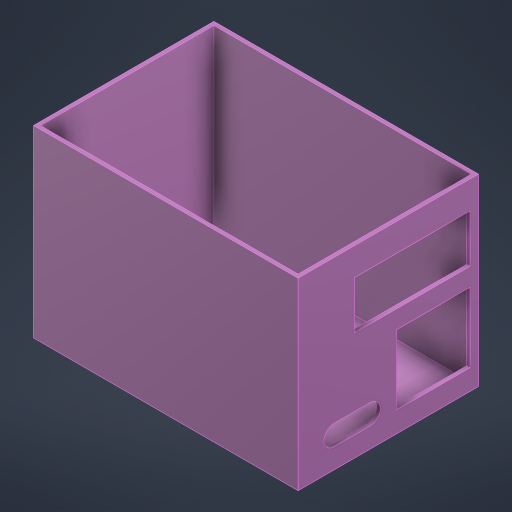
# Autodesk Inventor part: perspex_shell
Saved by Autodesk Inventor 2023 (Build 270158000, 158)
## iProperties
Created: 2022-11-19
Part Number: perspex_shell
Material: Generic
Document SubType Name: Modeling
Designer: washington
Density: 1 g/cm^3
Appearance: Smooth - Purple
Author: washington
Autodesk Inventor part; units mm, degrees
ref_plane "YZ Plane" through (0, 0, 0) normal (1, 0, 0) x (0, 1, 0)
ref_plane "XZ Plane" through (0, 0, 0) normal (0, 1, 0) x (-1, 0, 0)
ref_plane "XY Plane" through (0, 0, 0) normal (0, 0, 1) x (1, 0, 0)
sketch "Sketch1" plane through (0, 0, 0) normal (0, 1, 0) x (-1, 0, 0)
  line L0 (110, 75) -> (-110, 75)
  line L1 (-110, 75) -> (-110, -75)
  line L2 (-110, -75) -> (110, -75)
  line L3 (110, -75) -> (110, 75)
  line L4 (110, 75) -> (-110, -75) construction
  line L5 (-110, 75) -> (110, -75) construction
  point P0 (0, 0)
  dimension "d0" = 150
  dimension "d1" = 220
  constraints: 12 end point, 2 midpoint, 2 parallel, 1 horizontal, 1 perpendicular
  measures "d0" distance of L0.end L1.end
  measures "d1" distance of L1.end L2.end
extrude "Extrusion1" add sketch "Sketch1" along normal blind 3
sketch "Sketch2" plane through (0, 3, 0) normal (0, 1, 0) x (1, 0, 0)
  line L0 (110, -75) -> (110, 75) projected
  line L1 (-110, -75) -> (110, -75)
  line L2 (110, -75) -> (110, 75)
  line L3 (110, 75) -> (-110, 75)
  line L4 (-110, 75) -> (-110, -75)
  line L5 (-110, -75) -> (110, 75) construction
  line L6 (110, -75) -> (-110, 75) construction
  line L7 (-107, -72) -> (107, -72)
  line L8 (107, -72) -> (107, 72)
  line L9 (107, 72) -> (-107, 72)
  line L10 (-107, 72) -> (-107, -72)
  line L11 (-107, -72) -> (107, 72) construction
  line L12 (107, -72) -> (-107, 72) construction
  point P0 (0, 0)
  dimension "d4" = 144
  dimension "d5" = 214
  constraints: 24 end point, 4 midpoint, 4 parallel, 2 horizontal, 2 perpendicular
  measures "d4" distance of L7.end L8.end
  measures "d5" distance of L8.end L9.end
extrude "Extrusion2" add sketch "Sketch2" along normal blind 150
sketch "Sketch3" plane through (110, 0, 75) normal (1, 0, 0) x (0, 0, -1)
  line L0 (47, 130) -> (143, 130)
  line L1 (143, 130) -> (143, 90)
  line L2 (143, 90) -> (47, 90)
  line L3 (47, 90) -> (47, 130)
  line L4 (47, 130) -> (143, 90) construction
  line L5 (143, 130) -> (47, 90) construction
  line L6 (0, 0) -> (0, 153) projected
  line L7 (82, 75) -> (143, 75)
  line L8 (143, 75) -> (143, 17)
  line L9 (143, 17) -> (82, 17)
  line L10 (82, 17) -> (82, 75)
  line L11 (82, 75) -> (143, 17) construction
  line L12 (143, 75) -> (82, 17) construction
  line L13 (30, 25) -> (60, 25) construction
  line L14 (30, 16.456) -> (60, 16.456)
  line L15 (60, 33.544) -> (30, 33.544)
  arc A0 (30, 33.544) -> (30, 16.456) centre (30, 25) ccw
  arc A1 (60, 16.456) -> (60, 33.544) centre (60, 25) ccw
  point P0 (75, 0)
  point P1 (95, 110)
  point P2 (112.5, 46)
  point P3 (0, 3)
  point P4 (45, 25)
  dimension "d8" = 96
  dimension "d9" = 40
  dimension "d10" = 95
  dimension "d11" = 110
  dimension "d14" = 61
  dimension "d15" = 58
  dimension "d16" = 0
  dimension "d17" = 46
  dimension "d18" = 25
  dimension "d19" = 30
  dimension "d20" = 30
  dimension "d21" = 8.544
  constraints: 32 end point, 5 midpoint, 5 parallel, 4 point on circle, 4 tangent, 3 horizontal, 2 centre point, 2 perpendicular
  measures "d8" distance of L1.end L2.end
  measures "d9" distance of L0.end L1.end
  measures "d10" distance from line of point (95, 110) L6
  measures "d11" vertical distance of point (95, 110) L6.start
  measures "d14" distance of L8.end L9.end
  measures "d15" distance of L7.end L8.end
  measures "d16" distance between parallel lines of L1 L8
  measures "d17" vertical distance of L6.start point (112.5, 46)
  measures "d18" distance from line of L13 L6.start
  measures "d19" horizontal distance of L13.start L6.start
  measures "d20" distance of L13.start L13.end
  measures "d21" radius of A0
extrude "Extrusion3" cut sketch "Sketch3" against normal blind 3
body "Solid1"
